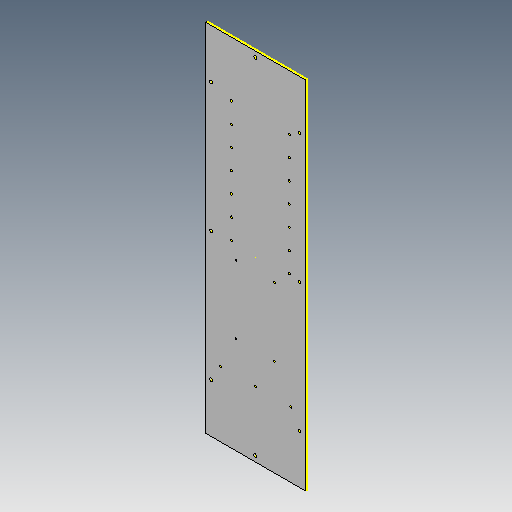
# Autodesk Inventor part: Cut_B
Saved by Autodesk Inventor 2020 (Build 240168000, 168)
## iProperties
Created: 2021-12-11
Part Number: Cut_B
Material: Generic
Document SubType Name: Modeling
Designer: magnarecta
Density: 1 g/cm^3
Appearance: Default
Author: magnarecta
Autodesk Inventor part; units mm, degrees
ref_plane "YZ Plane" through (0, 0, 0) normal (1, 0, 0) x (0, 1, 0)
ref_plane "XZ Plane" through (0, 0, 0) normal (0, 1, 0) x (-1, 0, 0)
ref_plane "XY Plane" through (0, 0, 0) normal (0, 0, 1) x (1, 0, 0)
sketch "スケッチ1" plane through (0, 0, 0) normal (0, 0, 1) x (1, 0, 0)
  line L0 (99, -354) -> (-99, -354)
  line L1 (-99, -354) -> (-99, 354)
  line L2 (-99, 354) -> (99, 354)
  line L3 (99, 354) -> (99, -354)
  line L4 (99, -354) -> (-99, 354) construction
  line L5 (-99, -354) -> (99, 354) construction
  point P0 (0, 0)
  dimension "d0" = 198
  dimension "d1" = 708
  constraints: 12 end point, 2 midpoint, 2 parallel, 1 horizontal, 1 perpendicular
  measures "d0" distance of L1.end L2.end
  measures "d1" distance of L0.end L1.end
extrude "押し出し1" add sketch "スケッチ1" along normal blind 3
sketch "スケッチ2" plane through (0, 0, 3) normal (0, 0, 1) x (1, 0, 0)
  line L0 (99, -354) -> (99, 354) projected
  line L1 (-99, -354) -> (99, -354) projected
  line L2 (99, 354) -> (-99, 354) projected
  point P0 (0, 0)
  point P1 (67.5, 244)
  point P2 (-47.5, 244)
  point P3 (67.5, 204)
  point P4 (-47.5, 204)
  point P5 (67.5, 164)
  point P6 (-47.5, 164)
  point P7 (67.5, 124)
  point P8 (-47.5, 124)
  point P9 (67.5, 84)
  point P10 (-47.5, 84)
  point P11 (67.5, 44)
  point P12 (-47.5, 44)
  point P13 (67.5, 4)
  point P14 (-47.5, 4)
  dimension "d4" = 115
  dimension "d7" = 40
  dimension "d12" = 47.5
  dimension "d21" = 110
  constraints: 1 horizontal alignment, 1 vertical, 12 other
  measures "d4" distance of point (67.5, 244) point (-47.5, 244)
  measures "d7" distance of point (67.5, 244) point (67.5, 204)
  measures "d12" horizontal distance of point (0, 0) point (-47.5, 244)
  measures "d21" distance from line of point (67.5, 244) L2
hole "穴1" at (67.5, 244, 3) at (-47.5, 244, 3) at (67.5, 204, 3) at (-47.5, 204, 3) at (67.5, 164, 3) at (-47.5, 164, 3) at (67.5, 124, 3) at (-47.5, 124, 3) at (67.5, 84, 3) at (-47.5, 84, 3) at (67.5, 44, 3) at (-47.5, 44, 3) at (67.5, 4, 3) at (-47.5, 4, 3) direction (0, 0, -1) diameter 4.2 end through all
sketch "スケッチ3" plane through (0, 0, 0) normal (0, 0, -1) x (-1, 0, 0)
  line L0 (38, -161) -> (-38, -161)
  line L1 (-38, -161) -> (-38, -26)
  line L2 (-38, -26) -> (38, -26)
  line L3 (38, -26) -> (38, -161)
  line L4 (38, -161) -> (-38, -26) construction
  line L5 (-38, -161) -> (38, -26) construction
  circle A0 centre (-67.5, 4) radius 2.1 projected
  circle A1 centre (-67.5, 44) radius 2.1 projected
  circle A2 centre (-67.5, 84) radius 2.1 projected
  circle A3 centre (-67.5, 124) radius 2.1 projected
  circle A4 centre (-67.5, 164) radius 2.1 projected
  circle A5 centre (-67.5, 204) radius 2.1 projected
  circle A6 centre (-67.5, 244) radius 2.1 projected
  circle A7 centre (47.5, 244) radius 2.1 projected
  circle A8 centre (47.5, 204) radius 2.1 projected
  circle A9 centre (47.5, 164) radius 2.1 projected
  circle A10 centre (47.5, 124) radius 2.1 projected
  circle A11 centre (47.5, 84) radius 2.1 projected
  circle A12 centre (47.5, 44) radius 2.1 projected
  circle A13 centre (47.5, 4) radius 2.1 projected
  line L6 (99, -354) -> (-99, -354) projected
  line L7 (99, 354) -> (99, -354) projected
  line L8 (-99, 354) -> (99, 354) projected
  line L9 (-99, -354) -> (-99, 354) projected
  point P0 (0, 0)
  point P1 (0, -93.5)
  point P2 (0, -93.5)
  dimension "d22" = 76
  dimension "d23" = 135
  dimension "d24" = 30
  constraints: 12 end point, 3 midpoint, 2 parallel, 1 horizontal, 1 perpendicular, 1 vertical alignment
  measures "d22" distance of L1.end L2.end
  measures "d23" distance of L0.end L1.end
  measures "d24" distance from line of A0.centre L2
hole "穴2" at (-38, -161, 0) at (38, -161, 0) at (38, -26, 0) at (-38, -26, 0) direction (0, 0, 1) diameter 3.5 end through all
sketch "スケッチ4" plane through (0, 0, 0) normal (0, 0, -1) x (-1, 0, 0)
  circle A0 centre (-38, -26) radius 1.75 projected
  circle A1 centre (38, -161) radius 1.75 projected
  circle A2 centre (-38, -161) radius 1.75 projected
  circle A3 centre (38, -26) radius 1.75 projected
  circle A4 centre (-67.5, 4) radius 2.1 projected
  circle A5 centre (-67.5, 44) radius 2.1 projected
  circle A6 centre (-67.5, 84) radius 2.1 projected
  circle A7 centre (-67.5, 124) radius 2.1 projected
  circle A8 centre (-67.5, 164) radius 2.1 projected
  circle A9 centre (-67.5, 204) radius 2.1 projected
  circle A10 centre (-67.5, 244) radius 2.1 projected
  circle A11 centre (47.5, 244) radius 2.1 projected
  circle A12 centre (47.5, 204) radius 2.1 projected
  circle A13 centre (47.5, 164) radius 2.1 projected
  circle A14 centre (47.5, 124) radius 2.1 projected
  circle A15 centre (47.5, 84) radius 2.1 projected
  circle A16 centre (47.5, 44) radius 2.1 projected
  circle A17 centre (47.5, 4) radius 2.1 projected
  line L0 (99, -354) -> (-99, -354) projected
  line L1 (99, 354) -> (99, -354) projected
  line L2 (-99, 354) -> (99, 354) projected
  line L3 (-99, -354) -> (-99, 354) projected
  line L4 (-88, 343) -> (88, 343)
  line L5 (88, 343) -> (88, -343)
  line L6 (88, -343) -> (-88, -343)
  line L7 (-88, -343) -> (-88, 343)
  line L8 (-88, -256.5) -> (88, -256.5)
  line L9 (88, -256.5) -> (88, 256.5)
  line L10 (88, 256.5) -> (-88, 256.5)
  line L11 (-88, 256.5) -> (-88, -256.5)
  point P0 (0, 0)
  point P1 (0, -343)
  point P2 (0, 343)
  point P3 (-88, 0)
  point P4 (88, 0)
  dimension "d32" = 11
  dimension "d33" = 86.5
  dimension "d34" = 86.5
  constraints: 16 end point, 4 midpoint, 2 parallel, 2 point on line, 1 horizontal, 1 perpendicular, 3 other
  measures "d32" distance between parallel lines of L3 L7
  measures "d33" distance from line of L8 point (0, -343)
  measures "d34" distance from line of point (0, 343) L10
hole "穴3" at (0, -343, 0) at (0, 343, 0) at (88, 0, 0) at (-88, 0, 0) at (-88, -256.5, 0) at (88, -256.5, 0) at (88, 256.5, 0) at (-88, 256.5, 0) direction (0, 0, 1) diameter 6 end through all
sketch "スケッチ5" plane through (0, 0, 0) normal (0, 0, -1) x (-1, 0, 0)
  line L0 (69.4488, -224) -> (-70.5512, -224)
  line L1 (99, -354) -> (-99, -354) projected
  point P0 (0, 0)
  point P1 (-0.5512, -224)
  dimension "d42" = 140
  dimension "d43" = 130
  constraints: 2 end point, 1 horizontal, 1 midpoint
  measures "d42" distance of L0.start L0.end
  measures "d43" distance between parallel lines of L0 L1
hole "穴4" at (0.5512, -224, 0) at (70.5512, -224, 0) at (-69.4488, -224, 0) direction (0, 0, 1) diameter 4.2 end through all
sketch "スケッチ6" plane through (0, 0, 0) normal (0, 0, -1) x (-1, 0, 0)
  circle A0 centre (-70.5512, -224) radius 2.1 projected
  circle A1 centre (-0.5512, -224) radius 2.1 projected
  circle A2 centre (69.4488, -224) radius 2.1 projected
  circle A3 centre (-88, 256.5) radius 3 projected
  circle A4 centre (88, -256.5) radius 3 projected
  circle A5 centre (-88, 0) radius 3 projected
  circle A6 centre (0, -343) radius 3 projected
  circle A7 centre (0, 343) radius 3 projected
  circle A8 centre (88, 0) radius 3 projected
  circle A9 centre (-88, -256.5) radius 3 projected
  circle A10 centre (88, 256.5) radius 3 projected
  circle A11 centre (-38, -26) radius 1.75 projected
  circle A12 centre (38, -161) radius 1.75 projected
  circle A13 centre (-38, -161) radius 1.75 projected
  circle A14 centre (38, -26) radius 1.75 projected
  circle A15 centre (-67.5, 4) radius 2.1 projected
  circle A16 centre (-67.5, 44) radius 2.1 projected
  circle A17 centre (-67.5, 84) radius 2.1 projected
  circle A18 centre (-67.5, 124) radius 2.1 projected
  circle A19 centre (-67.5, 164) radius 2.1 projected
  circle A20 centre (-67.5, 204) radius 2.1 projected
  circle A21 centre (-67.5, 244) radius 2.1 projected
  circle A22 centre (47.5, 244) radius 2.1 projected
  circle A23 centre (47.5, 204) radius 2.1 projected
  circle A24 centre (47.5, 164) radius 2.1 projected
  circle A25 centre (47.5, 124) radius 2.1 projected
  circle A26 centre (47.5, 84) radius 2.1 projected
  circle A27 centre (47.5, 44) radius 2.1 projected
  circle A28 centre (47.5, 4) radius 2.1 projected
  line L0 (99, -354) -> (-99, -354) projected
  line L1 (99, 354) -> (99, -354) projected
  line L2 (-99, 354) -> (99, 354) projected
  line L3 (-99, -354) -> (-99, 354) projected
  point P0 (0, 0)
